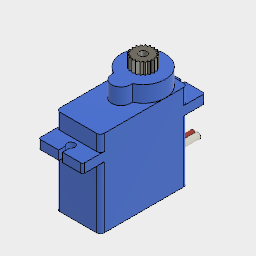
2941 Micro DC Motor (Autodesk Fusion 360 design; units mm, degrees)
Autodesk Fusion 360 part; units mm, degrees
note: some values were not read from the file. Set by a fixed rule: which sketch regions a step uses.
sketch "base" plane through (0, 0, 0) normal (0, 0, 1) x (1, 0, 0)
  line L0 (0, 0) -> (11.8, 0)
  line L1 (11.8, 0) -> (11.8, 23.2)
  line L2 (11.8, 23.2) -> (0, 23.2)
  line L3 (0, 23.2) -> (0, 0)
  dimension "d1" = 11.8
  dimension "d2" = 23.2
  measures "d1" distance of L0.start L0.end
  measures "d2" distance of L0.start L2.end
extrude "Extrude1" add sketch "base" along normal blind 16.4 makes body 1
sketch "tabs" plane through (0, 0, 16.4) normal (0, 0, 1) x (-1, 0, 0)
  line L0 (0, -23.2) -> (0, 0)
  line L1 (0, 0) -> (-11.8, 0)
  line L2 (-11.8, 0) -> (-11.8, -23.2)
  line L3 (-11.8, -23.2) -> (0, -23.2)
  line L4 (0, -11.6) -> (-11.8, -11.6) construction
  line L5 (-11.8, -27.9) -> (0, -27.9)
  line L6 (0, -27.9) -> (0, 4.7)
  line L7 (0, 4.7) -> (-11.8, 4.7)
  line L8 (-11.8, 4.7) -> (-11.8, -27.9)
  line L9 (-11.8, -27.9) -> (0, 4.7) construction
  line L10 (0, -27.9) -> (-11.8, 4.7) construction
  line L11 (-6.4, 2.766) -> (-6.4, 4.7)
  line L12 (-6.4, 4.7) -> (-5.4, 4.7)
  line L13 (-5.4, 4.7) -> (-5.4, 2.766)
  line L14 (-5.9, 1.9) -> (-5.9, 4.7) construction
  arc A0 (-6.4, 2.766) -> (-5.4, 2.766) centre (-5.9, 1.9) ccw
  arc A1 (-5.4, -25.966) -> (-6.4, -25.966) centre (-5.9, -25.1) ccw
  line L15 (-6.4, -25.966) -> (-6.4, -27.9)
  line L16 (-6.4, -27.9) -> (-5.4, -27.9)
  line L17 (-5.4, -27.9) -> (-5.4, -25.966)
  point P0 (-5.9, -11.6)
  dimension "d33" = 32.6
  dimension "d34" = 11.8
  dimension "d35" = 2
  dimension "d36" = 13.5
  dimension "d37" = 1
  measures "d33" distance of L5.end L6.end
  measures "d34" distance of L6.end L7.end
  measures "d35" diameter of A0
  measures "d36" distance of P0 L14.start
  measures "d37" distance of L11 L13
extrude "Extrude8" add sketch "tabs" along normal blind 2.4 contours L0 L1 L2 L3 L6 L8 | L3 L5 L6 L8 A1 L15 L17 | L1 L6 L7 L8 L11 L13 A0 bodies 1
extrude "Extrude9" add sketch "base" along normal blind 23 bodies 1
sketch "motor" plane through (0, 0, 23) normal (0, 0, 1) x (-1, 0, 0)
  line L0 (0, -23.2) -> (0, 0)
  line L1 (0, 0) -> (-11.8, 0)
  line L2 (-11.8, 0) -> (-11.8, -23.2)
  line L3 (-11.8, -23.2) -> (0, -23.2)
  circle A0 centre (-5.9, -17.3) radius 5.9
  circle A1 centre (-5.9, -11.4) radius 2.5
  dimension "d42" = 11.8
  dimension "d43" = 5
  measures "d42" diameter of A0
  measures "d43" diameter of A1
extrude "Extrude10" add sketch "motor" along normal blind 4.3 contours A0 A1 | A0 A1 | A0 A1 bodies 1
sketch "gear" plane through (0, 0, 27.3) normal (0, 0, 1) x (-1, 0, 0)
  arc A0 (-3.4568, -11.9297) -> (-8.3432, -11.9297) centre (-5.9, -11.4) ccw
  arc A1 (-8.3432, -11.9297) -> (-3.4568, -11.9297) centre (-5.9, -17.3) ccw
  circle A2 centre (-5.9, -17.3) radius 2.4
  circle A3 centre (-5.9, -17.3) radius 1
  dimension "d46" = 4.8
  dimension "d47" = 2
  measures "d46" diameter of A2
  measures "d47" diameter of A3
extrude "Extrude11" add sketch "gear" along normal blind 3 separate body contours A2 makes body 2
sketch "tooth" plane through (0, 0, 30.3) normal (0, 0, 1) x (-1, 0, 0)
  circle A0 centre (-5.9, -17.3) radius 1
  circle A1 centre (-5.9, -17.3) radius 2.4
  line L0 (-5.9, -17.3) -> (-5.9, -28.5) construction
  line L1 (-5.15, -19.3) -> (-6.65, -19.3)
  line L2 (-6.65, -19.3) -> (-5.9, -20.3)
  line L3 (-5.9, -20.3) -> (-5.15, -19.3)
  line L4 (-5.9, -20.3) -> (-5.9, -19.3) construction
  dimension "d50" = 1
  dimension "d51" = 1.5
  dimension "d56" = 2
  measures "d50" distance of L2.end L4.end
  measures "d51" distance of L1.start L1.end
  measures "d56" distance of A0.centre L1
extrude "Extrude12" add sketch "tooth" against normal up to surface (3 mm away) contours A1 L2 L3 bodies 2
pattern_circular "C-Pattern2" count 20 over 360 about axis through (5.9, 17.3, 30.3) along (0, 0, -1) of "Extrude12"
fillet "Fillet2" radius 1 8 edges at (11.8, 0, 20.9) (0, 0, 20.9) (11.8, 0, 8.2) (0, 0, 8.2) (11.8, 23.2, 8.2) (11.8, 23.2, 20.9) (0, 23.2, 20.9) (0, 23.2, 8.2) on bodies 1
fillet "Fillet3" radius 0.5 4 edges at (0, -4.7, 17.6) (11.8, -4.7, 17.6) (11.8, 27.9, 17.6) (0, 27.9, 17.6) on bodies 1
sketch "Sketch10" plane through (0, 23.2, 0) normal (0, 1, 0) x (-1, 0, 0)
  line L0 (-1, 0) -> (-1, 16.4)
  line L1 (-1, 16.4) -> (-10.8, 16.4)
  line L2 (-10.8, 16.4) -> (-10.8, 0)
  line L3 (-10.8, 0) -> (-1, 0)
  line L4 (-10.8, 4.8) -> (-1, 4.8) construction
  arc A0 (-5.95, 4.4258) -> (-5.95, 5.1742) centre (-5.3, 4.8) ccw
  arc A1 (-5.95, 5.1742) -> (-5.95, 4.4258) centre (-6.6, 4.8) ccw
  dimension "d59" = 4.8
  dimension "d60" = 1.5
  dimension "d61" = 1.5
  measures "d59" distance of L3 L4
  measures "d60" diameter of A1
  measures "d61" diameter of A0
extrude "Extrude13" add sketch "Sketch10" along normal blind 8 separate body contours A0 A1 makes body 3
equation "d36 = ( 27 / 2 ) * 1 mm"
equation "d46 = ( 2.4 * 2 ) * 1 mm"
